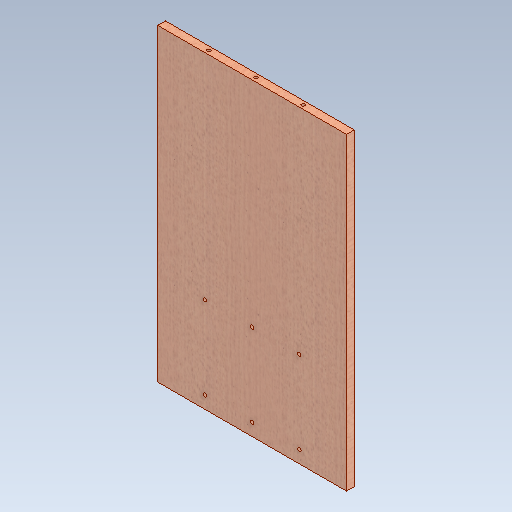
# Autodesk Inventor part: LateralInteriorPC
Saved by Autodesk Inventor 2020.3 (Build 243373000, 373)
## iProperties
Created: 2020-10-29
Part Number: LateralInteriorPC
Material: Madera (roble)
Document SubType Name: Modeling
Designer: codig
Density: 0.76 g/cm^3
Appearance: Roble blanco - Natural brillo medio
Author: codig
Autodesk Inventor part; units mm, degrees
ref_plane "YZ Plane" through (0, 0, 0) normal (1, 0, 0) x (0, 1, 0)
ref_plane "XZ Plane" through (0, 0, 0) normal (0, 1, 0) x (-1, 0, 0)
ref_plane "XY Plane" through (0, 0, 0) normal (0, 0, 1) x (1, 0, 0)
sketch "Boceto1" plane through (0, 0, 0) normal (0, 0, 1) x (1, 0, 0)
  line L0 (100, 100) -> (540, 100)
  line L1 (540, 100) -> (540, 820)
  line L2 (540, 820) -> (100, 820)
  line L3 (100, 820) -> (100, 100)
  point P0 (0, 0)
  constraints: 8 end point, 2 parallel, 1 horizontal, 1 perpendicular
extrude "Extrusión1" add sketch "Boceto1" along normal blind 18
sketch "Boceto2" plane through (100, 820, 0) normal (0, 1, 0) x (1, 0, 0)
  circle A0 centre (110, -9) radius 4
  circle A1 centre (220, -9) radius 4
  circle A2 centre (330, -9) radius 4
  point P0 (-100, 0)
  constraints: 3 centre point
hole "Agujero1" at (430, 820, 9) at (320, 820, 9) at (210, 820, 9) direction (0, -1, 0) diameter 8 depth 35
sketch "Boceto3" plane through (0, 0, 18) normal (0, 0, 1) x (1, 0, 0)
  circle A0 centre (430, 321) radius 4
  circle A1 centre (320, 321) radius 4
  circle A2 centre (210, 321) radius 4
  point P0 (0, 0)
  constraints: 3 centre point
hole "Agujero2" at (430, 321, 18) at (320, 321, 18) at (210, 321, 18) direction (0, 0, -1) diameter 8 depth 10
sketch "Boceto4" plane through (0, 0, 18) normal (0, 0, 1) x (1, 0, 0)
  line L0 (540, 100) -> (540, 820) projected
  circle A0 centre (210, 129) radius 4
  circle A1 centre (320, 129) radius 4
  circle A2 centre (430, 129) radius 4
  point P0 (0, 0)
  constraints: 3 centre point
hole "Agujero3" at (430, 129, 18) at (320, 129, 18) at (210, 129, 18) direction (0, 0, -1) diameter 8 depth 10
sketch "Boceto5" plane through (100, 100, 0) normal (0, -1, 0) x (1, 0, 0)
  circle A0 centre (330, 9) radius 4
  circle A1 centre (220, 9) radius 4
  circle A2 centre (110, 9) radius 4
  point P0 (-100, 0)
  constraints: 3 centre point
hole "Agujero4" at (430, 100, 9) at (320, 100, 9) at (210, 100, 9) direction (0, 1, 0) diameter 8 depth 23
